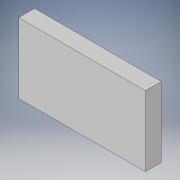
# Autodesk Inventor part: Convex Organ Bank Joint Slot
Saved by Autodesk Inventor 2019 (Build 230136000, 136)
## iProperties
Created: 2021-02-18
Part Number: Convex Organ Bank Joint Slot
Material: Generic
Document SubType Name: Modeling
Designer: Eric
Density: 1 g/cm^3
Appearance: Default
Author: Eric
Autodesk Inventor part; units mm, degrees
ref_plane "YZ Plane" through (0, 0, 0) normal (1, 0, 0) x (0, 1, 0)
ref_plane "XZ Plane" through (0, 0, 0) normal (0, 1, 0) x (-1, 0, 0)
ref_plane "XY Plane" through (0, 0, 0) normal (0, 0, 1) x (1, 0, 0)
sketch "Sketch1" plane through (0, 0, 0) normal (0, 0, 1) x (1, 0, 0)
  line L0 (0, 0) -> (95.159, 0)
  line L1 (95.159, 0) -> (95.159, -52.6)
  line L2 (95.159, -52.6) -> (0, -52.6)
  line L3 (0, -52.6) -> (0, 0)
  dimension "d0" = 52.6
  dimension "d1" = 95.159
  constraints: 8 end point, 2 horizontal, 1 vertical
  measures "d0" distance of L0.end L1.end
  measures "d1" distance between parallel lines of L1 L3
extrude "Extrusion1" add sketch "Sketch1" along normal blind 12
body "Solid1"
